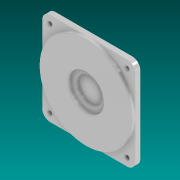
# Autodesk Inventor part: base onderkant
Saved by Autodesk Inventor 2020.2 (Build 242310000, 310)
## iProperties
Created: 2020-05-19
Part Number: base onderkant
Material: Aluminum 6061
Document SubType Name: Modeling
Designer: Svend
Density: 2.7 g/cm^3
Appearance: Aluminum - Polished
Author: Svend
Autodesk Inventor part; units mm, degrees
ref_plane "YZ Plane" through (0, 0, 0) normal (1, 0, 0) x (0, 1, 0)
ref_plane "XZ Plane" through (0, 0, 0) normal (0, 1, 0) x (-1, 0, 0)
ref_plane "XY Plane" through (0, 0, 0) normal (0, 0, 1) x (1, 0, 0)
sketch "Sketch1" plane through (0, 0, 0) normal (0, 0, 1) x (1, 0, 0)
  circle A0 centre (0, 0) radius 90
  circle A1 centre (0, 0) radius 35
  line L0 (-75, 90) -> (75, 90)
  line L1 (90, 75) -> (90, -75)
  line L2 (75, -90) -> (-75, -90)
  line L3 (-90, -75) -> (-90, 75)
  line L4 (-90, 90) -> (90, -90) construction
  line L5 (90, 90) -> (-90, -90) construction
  arc A2 (-75, 90) -> (-90, 75) centre (-75, 75) ccw
  arc A3 (90, 75) -> (75, 90) centre (75, 75) ccw
  arc A4 (75, -90) -> (90, -75) centre (75, -75) ccw
  arc A5 (-90, -75) -> (-75, -90) centre (-75, -75) ccw
  circle A6 centre (75, 75) radius 4.25
  circle A7 centre (75, -75) radius 4.25
  circle A8 centre (-75, -75) radius 4.25
  circle A9 centre (-75, 75) radius 4.25
  point P0 (0, 90)
  point P1 (90, 0)
  point P2 (0, -90)
  point P3 (-90, 0)
  dimension "d0" = 180
  dimension "d1" = 70
  dimension "d2" = 15
  dimension "d3" = 8.5
  constraints: 12 end point, 10 centre point, 10 tangent, 8 point on circle, 8 point on line, 6 coincident, 6 equal radius, 2 midpoint, 2 parallel, 1 horizontal, 1 perpendicular
  measures "d0" diameter of A0
  measures "d1" diameter of A1
  measures "d2" radius of A2
  measures "d3" diameter of A6
extrude "Extrusion1" add sketch "Sketch1" along normal blind 10 contours A0 | A1
extrude "Extrusion2" add sketch "Sketch1" along normal blind 5 contours L1 A4 L2 A0 | A0 L0 A3 L1 | A0 L3 A2 L0 | L2 A5 L3 A0
sketch "Sketch2" plane through (0, 0, 10) normal (0, 0, 1) x (1, 0, 0)
  circle A0 centre (0, 0) radius 35
  dimension "d8" = 70
  constraints: 1 centre point, 1 coincident
  measures "d8" diameter of A0
extrude "Extrusion3" cut sketch "Sketch2" against normal blind 6.5
sketch "Sketch3" plane through (0, 0, 0) normal (0, 0, -1) x (-1, 0, 0)
  circle A0 centre (-75, 75) radius 4.25 projected
  circle A1 centre (75, 75) radius 4.25 projected
  circle A2 centre (-75, -75) radius 4.25 projected
  circle A3 centre (75, -75) radius 4.25 projected
  line L0 (-90, -75) -> (-90, 75) projected
  arc A4 (-90, -75) -> (-75, -90) centre (-75, -75) ccw projected
  line L1 (75, -90) -> (-75, -90) projected
  arc A5 (75, -90) -> (90, -75) centre (75, -75) ccw projected
  line L2 (90, 75) -> (90, -75) projected
  arc A6 (90, 75) -> (75, 90) centre (75, 75) ccw projected
  line L3 (-75, 90) -> (75, 90) projected
  arc A7 (-75, 90) -> (-90, 75) centre (-75, 75) ccw projected
  point P0 (0, 0)
extrude "Extrusion4" add sketch "Sketch3" along normal blind 5
sketch "Sketch4" plane through (0, 0, 3.5) normal (0, 0, 1) x (1, 0, 0)
  circle A0 centre (0, 0) radius 35 projected
  circle A1 centre (0, 0) radius 25
  dimension "d13" = 50
  constraints: 1 centre point, 1 coincident
  measures "d13" diameter of A1
extrude "Extrusion5" cut sketch "Sketch4" against normal blind 5 contours A1
body "Solid1"
